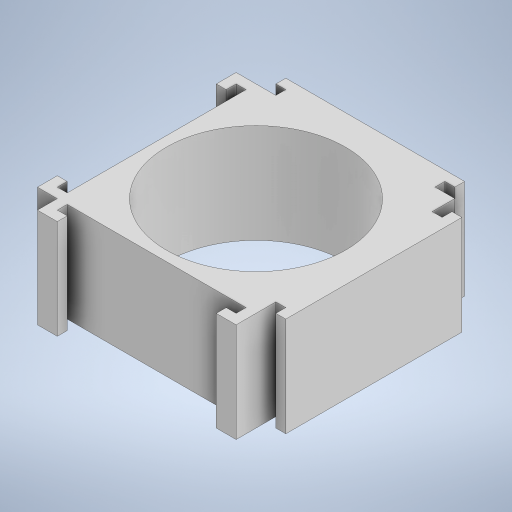
# Autodesk Inventor part: Maschio-femmina
Saved by Autodesk Inventor 2024 (Build 280153000, 153)
## iProperties
Created: 2024-01-14
Part Number: Maschio-femmina
Material: Generico
Document SubType Name: Modeling
Designer: Leonardo
Density: 1 g/cm^3
Appearance: Default
Author: Leonardo
Autodesk Inventor part; units mm, degrees
ref_plane "YZ Plane" through (0, 0, 0) normal (1, 0, 0) x (0, 1, 0)
ref_plane "XZ Plane" through (0, 0, 0) normal (0, 1, 0) x (-1, 0, 0)
ref_plane "XY Plane" through (0, 0, 0) normal (0, 0, 1) x (1, 0, 0)
sketch "Schizzo1" plane through (0, 0, 0) normal (0, 1, 0) x (-1, 0, 0)
  circle A0 centre (0, 0) radius 9
  line L0 (10, -10) -> (9, -10)
  line L1 (-10, 9) -> (-10, 10)
  line L2 (10, 10) -> (12, 10)
  line L3 (12, 10) -> (12, 9)
  line L4 (11, 9) -> (11, 8)
  line L5 (11, 8) -> (12, 8)
  line L6 (12, 8) -> (12, 9)
  line L7 (11, 9) -> (10, 9)
  line L8 (10, -10) -> (12, -10)
  line L9 (12, -10) -> (12, -9)
  line L10 (11, -9) -> (11, -8)
  line L11 (11, -8) -> (12, -8)
  line L12 (12, -8) -> (12, -9)
  line L13 (11, -9) -> (10, -9)
  line L14 (10, 9) -> (10, -9)
  line L15 (-9, 12) -> (-10, 12)
  line L16 (-10, 12) -> (-10, 10)
  line L17 (-9, 12) -> (-8, 12)
  line L18 (-8, 12) -> (-8, 11)
  line L19 (-8, 11) -> (-9, 11)
  line L20 (-9, 11) -> (-9, 10)
  line L21 (9, 12) -> (10, 12)
  line L22 (10, 12) -> (10, 10)
  line L23 (9, 12) -> (8, 12)
  line L24 (8, 12) -> (8, 11)
  line L25 (8, 11) -> (9, 11)
  line L26 (9, 11) -> (9, 10)
  line L27 (9, 10) -> (-9, 10)
  line L28 (-10, -10.0148) -> (-9, -10.0148)
  line L29 (9, -10) -> (8, -10)
  line L30 (-9, -10.0148) -> (-8, -10.0148)
  line L31 (-8, -10.0148) -> (-8, -11.0148)
  line L32 (-8, -11.0148) -> (-9, -11.0148)
  line L33 (-9, -11.0148) -> (-9, -12)
  line L34 (8, -10) -> (8, -11)
  line L35 (8, -11) -> (9, -11)
  line L36 (9, -11) -> (9, -12)
  line L37 (9, -12) -> (-9, -12)
  line L38 (-10, 9) -> (-10, 8)
  line L39 (-10, 8) -> (-11, 8)
  line L40 (-11, 8) -> (-11, 9)
  line L41 (-11, 9) -> (-12, 9)
  line L42 (-10, -10.0148) -> (-10, -7.7324)
  line L43 (-10, -7.7324) -> (-11, -7.7324)
  line L44 (-11, -7.7324) -> (-11, -8.7324)
  line L45 (-11, -8.7324) -> (-12, -8.7324)
  line L46 (-12, -8.7324) -> (-12, 9)
  dimension "d0" = 18
  dimension "d16" = 2
  dimension "d17" = 1
  dimension "d18" = 1
  dimension "d19" = 1
  dimension "d20" = 2
  dimension "d21" = 1
  dimension "d22" = 1
  dimension "d23" = 1
  dimension "d24" = 1
  dimension "d26" = 1
  dimension "d27" = 2
  dimension "d28" = 1
  dimension "d29" = 1
  dimension "d30" = 1
  dimension "d36" = 1
  dimension "d37" = 1
  dimension "d38" = 1
  dimension "d39" = 1
  dimension "d40" = 1
  constraints: 94 end point, 17 perpendicular, 11 horizontal, 6 vertical, 4 parallel, 1 centre point, 1 coincident
  measures "d0" diameter of A0
  measures "d16" distance of L3.end L7.end
  measures "d17" distance of L2.end L3.end
  measures "d18" distance of L5.end L4.end
  measures "d19" distance of L4.end L4.start
  measures "d20" distance of L13.end L9.end
  measures "d21" distance of L9.end L8.end
  measures "d22" distance of L10.end L11.end
  measures "d23" distance of L10.start L10.end
  measures "d24" distance of L10.start L13.end
  measures "d26" distance of L15.end L15.start
  measures "d27" distance of L15.start L20.end
  measures "d28" distance of L18.end L19.end
  measures "d29" distance of L17.end L18.end
  measures "d30" distance of L25.end L24.end
  measures "d36" distance of L0.end L29.end
  measures "d37" distance of L30.end L31.end
  measures "d38" distance of L35.end L36.end
  measures "d39" distance of L40.end L41.end
  measures "d40" distance of L43.end L44.end
extrude "Estrusione2" add sketch "Schizzo1" along normal blind 10
